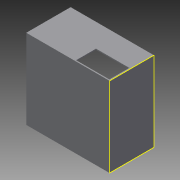
# Autodesk Inventor part: Case
Saved by Autodesk Inventor 2014 SP1 (Build 180222100, 222)
## iProperties
Created: 2014-11-08
Part Number: Case
Material: Generic
Document SubType Name: Modeling
Designer: Alex
Density: 1 g/cm^3
Appearance: Default
Author: Alex
Autodesk Inventor part; units mm, degrees
ref_plane "YZ Plane" through (0, 0, 0) normal (1, 0, 0) x (0, 1, 0)
ref_plane "XZ Plane" through (0, 0, 0) normal (0, 1, 0) x (-1, 0, 0)
ref_plane "XY Plane" through (0, 0, 0) normal (0, 0, 1) x (1, 0, 0)
sketch "Sketch1" plane through (0, 0, 0) normal (0, 1, 0) x (-1, 0, 0)
  line L0 (0, 0) -> (125, 0)
  line L1 (125, 0) -> (125, 120)
  line L2 (125, 120) -> (0, 120)
  line L3 (0, 120) -> (0, 0)
  dimension "d0" = 125
  dimension "d1" = 120
  constraints: 8 end point, 2 parallel, 1 horizontal, 1 perpendicular
  measures "d0" distance of L2.end L1.end
  measures "d1" distance of L1.end L0.end
extrude "Extrusion1" add sketch "Sketch1" along normal blind 1.75
sketch "Sketch2" plane through (0, 1.75, 0) normal (0, 1, 0) x (1, 0, 0)
  line L0 (0, 0) -> (-125, 0) projected
  line L1 (-125, 0) -> (-125, -120) projected
  line L2 (-125, -120) -> (0, -120) projected
  line L3 (0, -120) -> (0, 0) projected
  line L4 (-125, 0) -> (-119.2077, 0)
  line L5 (-125, -4.4946) -> (-125, 0)
  line L6 (-125, 0) -> (-123.25, 0)
  line L7 (-123.25, 0) -> (-123.25, -1.75)
  line L8 (-123.25, -1.75) -> (-125, -1.75)
  line L9 (-125, -1.75) -> (-125, 0)
  line L10 (0, -120) -> (-1.75, -120)
  line L11 (-1.75, -120) -> (-1.75, -118.25)
  line L12 (-1.75, -118.25) -> (0, -118.25)
  line L13 (0, -118.25) -> (0, -120)
  line L14 (-1.75, -118.25) -> (-123.25, -118.25)
  line L15 (-123.25, -118.25) -> (-123.25, -1.75)
  line L16 (-123.25, -1.75) -> (-1.75, -1.75)
  line L17 (-1.75, -1.75) -> (-1.75, -118.25)
  dimension "d4" = 1.75
  dimension "d5" = 1.75
  dimension "d6" = 1.75
  dimension "d7" = 1.75
  constraints: 28 end point, 6 parallel, 4 horizontal, 3 perpendicular
  measures "d4" distance of L7.end L8.end
  measures "d5" distance of L6.end L7.end
  measures "d6" distance of L11.end L12.end
  measures "d7" distance of L10.end L11.end
extrude "Extrusion2" add sketch "Sketch2" along normal blind 65 contours L3 L12 L17 L16 L7 L0 | L3 L2 L11 L12 | L7 L8 L1 L0 | L11 L2 L1 L8 L15 L14
sketch "Sketch3" plane through (0, 0, 120) normal (1, 0, 0) x (0, 0, -1)
  line L0 (0, 0) -> (120, 0) projected
  line L1 (120, 0) -> (120, 66.75) projected
  line L2 (0, 66.75) -> (120, 66.75) projected
  line L3 (0, 0) -> (0, 66.75) projected
sketch "Sketch4" plane through (0, 0, 0) normal (0, 0, -1) x (-1, 0, 0)
  line L0 (0, 0) -> (1.75, 0)
  line L1 (1.75, 0) -> (1.75, 30)
  line L2 (1.75, 30) -> (0, 30)
  line L3 (0, 30) -> (0, 0)
  line L4 (1.75, 30) -> (16.75, 30)
  line L5 (16.75, 30) -> (16.75, 0)
  line L6 (16.75, 0) -> (1.75, 0)
  line L7 (1.75, 0) -> (1.75, 30)
  line L8 (0, 0) -> (55, 0)
  line L9 (55, 0) -> (55, 1.75)
  line L10 (55, 1.75) -> (0, 1.75)
  line L11 (0, 1.75) -> (0, 0)
  line L12 (16.75, 1.75) -> (46.75, 1.75)
  line L13 (46.75, 1.75) -> (46.75, 30)
  line L14 (46.75, 30) -> (16.75, 30)
  line L15 (16.75, 30) -> (16.75, 1.75)
  dimension "d10" = 1.75
  dimension "d11" = 30
  dimension "d12" = 15
  dimension "d13" = 30
  dimension "d14" = 55
  dimension "d15" = 1.75
  dimension "d16" = 30
  constraints: 32 end point, 8 parallel, 4 horizontal, 4 perpendicular, 2 point on line
  measures "d10" distance of L2.end L1.end
  measures "d11" distance of L1.end L0.end
  measures "d12" distance of L5.end L6.end
  measures "d13" distance of L4.end L5.end
  measures "d14" distance of L10.end L9.end
  measures "d15" distance of L9.end L8.end
  measures "d16" distance of L14.end L13.end
extrude "Extrusion3" cut sketch "Sketch4" against normal blind 4 contours L5 L14 L13 L10
sketch "Sketch5" plane through (-125, 0, 120) normal (0, 0, 1) x (1, 0, 0)
  line L0 (125, 0) -> (125, 66.75) projected
  line L1 (0, 66.75) -> (125, 66.75) projected
  line L2 (0, 0) -> (125, 0)
  line L3 (125, 0) -> (125, 1.75)
  line L4 (125, 1.75) -> (0, 1.75)
  line L5 (0, 1.75) -> (0, 0)
  line L6 (125, 1.75) -> (123.25, 1.75)
  line L7 (123.25, 1.75) -> (123.25, 66.75)
  line L8 (123.25, 66.75) -> (125, 66.75)
  line L9 (125, 66.75) -> (125, 1.75)
  line L10 (123.25, 1.75) -> (73.25, 1.75)
  line L11 (73.25, 1.75) -> (73.25, 31.75)
  line L12 (73.25, 31.75) -> (123.25, 31.75)
  line L13 (123.25, 31.75) -> (123.25, 1.75)
  dimension "d19" = 1.75
  dimension "d20" = 1.75
  dimension "d21" = 50
  dimension "d22" = 30
  constraints: 24 end point, 6 parallel, 3 horizontal, 3 perpendicular, 2 point on line
  measures "d19" distance of L3.end L2.end
  measures "d20" distance of L7.end L8.end
  measures "d21" distance of L11.end L12.end
  measures "d22" distance of L10.end L11.end
extrude "Extrusion4" cut sketch "Sketch5" against normal blind 8621077.25 contours L4 L11 L12 L7
body "Solid1"
